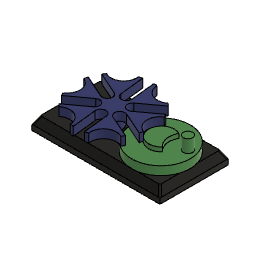
mechanism (Autodesk Fusion 360 design; units mm, degrees)
Autodesk Fusion 360 part; units mm, degrees
sketch "holder" plane through (0, 0, 0) normal (0, 0, 1) x (1, 0, 0)
  line L0 (0, 80) -> (150, 80)
  line L1 (150, 80) -> (150, 0)
  line L2 (150, 0) -> (0, 0)
  line L3 (0, 0) -> (0, 80)
  constraint horizontal L0
  constraint vertical L1
  constraint horizontal L2
  constraint vertical L3
extrude "Extrude1" add sketch "holder" along normal blind 15 makes body 1
chamfer "Chamfer1" distance 5 angle 60 4 edges at (150, 40, 15) (75, 0, 15) (0, 40, 15) (75, 80, 15) measured on face at (50, 53.3333, 15) measured on face at (50, 53.3333, 15) measured on face at (50, 53.3333, 15) measured on face at (50, 53.3333, 15) on bodies 1
fillet "Fillet1" radius 2 4 edges at (147.5, 2.5, 10.6699) (2.5, 2.5, 10.6699) (147.5, 77.5, 10.6699) (2.5, 77.5, 10.6699) on bodies 1
sketch "crank" plane through (0, 0, 15) normal (0, 0, 1) x (-1, 0, 0)
  ellipse E0 centre (-7.3094, -72.6906) end of major axis (-5.4837, -74.5163) minor radius 2 (-6.7321, -75) -> (-5, -73.2679) ccw
  line L0 (-5, -73.2679) -> (-5, -6.7321)
  ellipse E1 centre (-7.3094, -7.3094) end of major axis (-5.4837, -5.4837) minor radius 2 (-5, -6.7321) -> (-6.7321, -5) ccw
  line L1 (-6.7321, -5) -> (-143.2679, -5)
  ellipse E2 centre (-142.6906, -7.3094) end of major axis (-144.5163, -5.4837) minor radius 2 (-143.2679, -5) -> (-145, -6.7321) ccw
  line L2 (-145, -6.7321) -> (-145, -73.2679)
  ellipse E3 centre (-142.6906, -72.6906) end of major axis (-144.5163, -74.5163) minor radius 2 (-145, -73.2679) -> (-143.2679, -75) ccw
  line L3 (-143.2679, -75) -> (-6.7321, -75)
  circle A0 centre (-110.6408, -40) radius 34.3592
  constraint tangent L2 A0
extrude "Extrude2" add sketch "crank" along normal blind 10 separate body contours A0 makes body 2
sketch "moon?" plane through (0, 0, 25) normal (0, 0, 1) x (-1, 0, 0)
  circle A0 centre (-110.6408, -40) radius 34.3592
  circle A1 centre (-111.2844, -40.4363) radius 15
  circle A2 centre (-127.8196, -23.4394) radius 18.6957
  dimension "d9" = 30
  measures "d9" diameter of A1
extrude "Extrude3" add sketch "moon?" along normal blind 5 contours A1 A2 picked at (-112.2493, -43.1648) bodies 2
move_body "Move1" bodies 2 to x (1, 0, 0) y (0, 1, 0) z (0, 0, 1) at (0.8845, -0.7411, 0)
sketch "pin" plane through (0, 0, 25) normal (0, 0, 1) x (-1, 0, 0)
  circle A0 centre (-111.5252, -39.2589) radius 34.3592
  circle A1 centre (-131.401, -23.8792) radius 5.5042
  arc A2 (-127.0802, -41.3233) -> (-110.1308, -24.8343) centre (-128.704, -22.6983) ccw
  arc A3 (-127.0802, -41.3233) -> (-110.1308, -24.8343) centre (-112.1688, -39.6952) ccw
extrude "Extrude4" add sketch "pin" along normal blind 15 contours A1 bodies 2
move_body "Move2" bodies 2 to x (-0.866025, -0.5, 0) y (0.5, -0.866025, 0) z (0, 0, 1) at (189.4623, 130.1567, 0)
sketch "star" plane through (0, 0, 25) normal (0, 0, 1) x (-1, 0, 0)
  circle A0 centre (-87.6053, -43.7762) radius 5.5042
  arc A1 (-100.0693, -30.8295) -> (-106.5034, -53.5841) centre (-89.3504, -46.1473) ccw
  arc A2 (-100.0693, -30.8295) -> (-106.5034, -53.5841) centre (-112.1688, -39.6952) ccw
  circle A3 centre (-112.508, -40.3948) radius 34.3592
  circle A4 centre (-50, -40) radius 45.2769
  line L0 (-66.8993, -35.7179) -> (-97.8023, -40.3394)
  arc A5 (-97.8023, -40.3394) -> (-96.0275, -52.2074) centre (-96.9149, -46.2734) ccw
  line L1 (-96.0275, -52.2074) -> (-65.1245, -47.586)
  arc A6 (-65.1245, -47.586) -> (-66.8993, -35.7179) centre (-66.0119, -41.6519) ccw
  line L2 (-60.0779, -40.7645) -> (-102.8489, -47.1608) construction
  line L3 (-62.4418, -85.9647) -> (-50.9926, -56.8912)
  line L4 (-62.1581, -52.4942) -> (-73.6072, -81.5677)
  arc A7 (-50.9926, -56.8912) -> (-62.1581, -52.4942) centre (-56.5753, -54.6927) ccw
  arc A8 (-73.6072, -81.5677) -> (-62.4418, -85.9647) centre (-68.0245, -83.7662) ccw
  line L5 (-16.4143, -73.7573) -> (-35.8681, -49.3052)
  line L6 (-45.2587, -56.7763) -> (-25.8049, -81.2283)
  arc A9 (-35.8681, -49.3052) -> (-45.2587, -56.7763) centre (-40.5634, -53.0408) ccw
  arc A10 (-25.8049, -81.2283) -> (-16.4143, -73.7573) centre (-21.1096, -77.4928) ccw
  line L7 (-3.9725, -27.7926) -> (-34.8755, -32.414)
  line L8 (-33.1007, -44.2821) -> (-2.1977, -39.6606)
  arc A11 (-34.8755, -32.414) -> (-33.1007, -44.2821) centre (-33.9881, -38.3481) ccw
  arc A12 (-2.1977, -39.6606) -> (-3.9725, -27.7926) centre (-3.0851, -33.7266) ccw
  line L9 (-37.5582, 5.9647) -> (-49.0074, -23.1088)
  line L10 (-37.8419, -27.5058) -> (-26.3928, 1.5677)
  arc A13 (-49.0074, -23.1088) -> (-37.8419, -27.5058) centre (-43.4247, -25.3073) ccw
  arc A14 (-26.3928, 1.5677) -> (-37.5582, 5.9647) centre (-31.9755, 3.7662) ccw
  line L11 (-83.5857, -6.2427) -> (-64.1319, -30.6948)
  line L12 (-54.7413, -23.2237) -> (-74.1951, 1.2283)
  arc A15 (-64.1319, -30.6948) -> (-54.7413, -23.2237) centre (-59.4366, -26.9592) ccw
  arc A16 (-74.1951, 1.2283) -> (-83.5857, -6.2427) centre (-78.8904, -2.5072) ccw
  arc A17 (-32.1068, -99.4402) -> (-53.0309, -101.0083) centre (-43.37, -89.5337) ccw
  arc A18 (10.4233, -54.2241) -> (1.3193, -73.129) centre (-3.7876, -59.0251) ccw
  arc A19 (-7.4699, 5.2161) -> (4.3502, -12.1207) centre (-10.4176, -9.4914) ccw
  arc A20 (-67.8932, 19.4402) -> (-46.9691, 21.0083) centre (-56.63, 9.5337) ccw
  arc A21 (-110.4233, -25.7759) -> (-101.3193, -6.871) centre (-96.2124, -20.9749) ccw
  arc A22 (-92.5301, -85.2161) -> (-104.3502, -67.8793) centre (-89.5824, -70.5086) ccw
  dimension "d14" = 12
  dimension "d16" = 360
  dimension "d18" = 360
  constraint tangent L0 A5
  constraint tangent A5 L1
  constraint parallel L0 L1
  constraint tangent L1 A6
  constraint tangent L0 A6
  constraint midpoint A6 L2.start
  constraint midpoint A5 L2.end
  measures "d14" diameter of A5
extrude "Extrude5" add sketch "star" along normal blind 10 separate body contours A0 L0 | A0 A3 A4 L0 A21 | A3 A4 L0 L1 A6 L3 L4 A7 L5 L6 A9 L7 L8 A11 L9 L10 A13 L11 L12 A15 A17 A18 A19 A20 A21 A22 | A3 A4 L1 A22 picked at (-87.7474, -38.7381) makes body 3
move_body "Move3" bodies 3 to x (0.999391, -0.034899, 0) y (0.034899, 0.999391, 0) z (0, 0, 1) at (-1.3655, 1.7693, 0)
sketch "star stand" plane through (0, 0, 15) normal (0, 0, 1) x (-1, 0, 0)
  ellipse E0 centre (-7.3094, -72.6906) end of major axis (-5.4837, -74.5163) minor radius 2 (-6.7321, -75) -> (-5, -73.2679) ccw
  line L0 (-5, -73.2679) -> (-5, -6.7321)
  ellipse E1 centre (-7.3094, -7.3094) end of major axis (-5.4837, -5.4837) minor radius 2 (-5, -6.7321) -> (-6.7321, -5) ccw
  line L1 (-6.7321, -5) -> (-143.2679, -5)
  ellipse E2 centre (-142.6906, -7.3094) end of major axis (-144.5163, -5.4837) minor radius 2 (-143.2679, -5) -> (-145, -6.7321) ccw
  line L2 (-145, -6.7321) -> (-145, -73.2679)
  ellipse E3 centre (-142.6906, -72.6906) end of major axis (-144.5163, -74.5163) minor radius 2 (-145, -73.2679) -> (-143.2679, -75) ccw
  line L3 (-143.2679, -75) -> (-6.7321, -75)
  circle A0 centre (-50, -40) radius 10
extrude "Extrude6" add sketch "star stand" along normal blind 10 contours A0 bodies 3
move_body "Move4" bodies 3 to x (1, 0, 0) y (0, 1, 0) z (0, 0, 1) at (6.4578, 0.8932, 0)
move_body "Move5" bodies 2 to x (-0.965926, -0.258819, 0) y (0.258819, -0.965926, 0) z (0, 0, 1) at (210.2417, 107.0692, 0)
move_body "Move6" bodies 3 to x (0.906308, 0.422618, 0) y (-0.422618, 0.906308, 0) z (0, 0, 1) at (25.9343, -21.7099, 0)
copy_body "Body->Comp1" bodies 1 removing the originals makes body 4 in component "holder"
copy_body "Body->Comp2" bodies 2 removing the originals makes body 5 in component "crank"
copy_body "Body->Comp3" bodies 3 removing the originals makes body 6 in component "slot star"
move_body "Move1'" bodies 6 to x (1, 0, 0) y (0, 1, 0) z (0, 0, 1) at (-1.3067, -1.4628, 0) in component "slot star"
move_body "Move2'" bodies 6 to x (1, 0, 0) y (0, 1, 0) z (0, 0, 1) at (-1.4337, 0.9216, 0) in component "slot star"
component "holder" placed x (1, 0, 0) y (0, 1, 0) z (0, 0, 1) at (0, 0, 0)
component "crank" placed x (1, 0, 0) y (0, 1, 0) z (0, 0, 1) at (0, 0, 0)
component "slot star" placed x (1, 0, 0) y (0, 1, 0) z (0, 0, 1) at (0, 0, 0)
named bodies: "holder body", "crank body", "slot star body"
